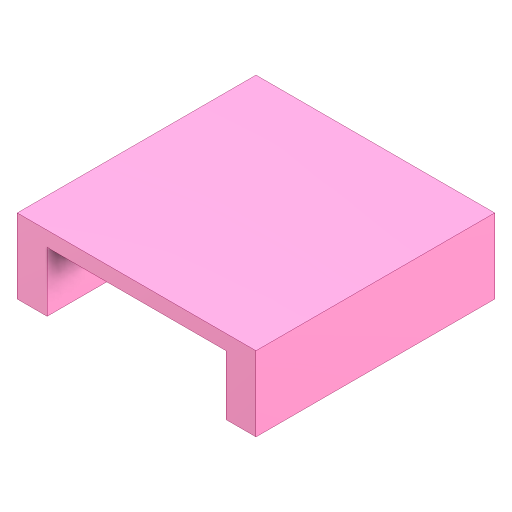
# Autodesk Inventor part: bridge_rect_final_12
Saved by Autodesk Inventor 2024 (Build 280153000, 153)
## iProperties
Created: 2023-08-28
Part Number: bridge_rect_final_12
Material: 一般
Document SubType Name: Modeling
Designer: admin
Density: 1 g/cm^3
Appearance: 平滑 - 白色
Author: admin
Autodesk Inventor part; units mm, degrees
sketch "草圖2" plane through (0, 0, 0) normal (0, 0, 1) x (1, 0, 0)
  line L0 (0, 30) -> (0, 0)
  line L1 (0, 0) -> (12, 0)
  line L2 (12, 0) -> (12, 24)
  line L3 (12, 24) -> (84, 24)
  line L4 (84, 24) -> (84, 0)
  line L5 (84, 0) -> (96, 0)
  line L6 (96, 0) -> (96, 30)
  line L7 (96, 30) -> (0, 30)
  dimension "d11" = 12
  dimension "d12" = 6
  dimension "d14" = 96
  dimension "d17" = 24
  constraints: 16 end point, 3 vertical, 2 collinear, 2 horizontal, 2 perpendicular, 1 coincident, 1 parallel
  measures "d11" distance of L0.end L1.end
  measures "d12" distance between parallel lines of L3 L7
  measures "d14" distance of L6.end L0.start
  measures "d17" distance between parallel lines of L1 L3
extrude "擠出2" add sketch "草圖2" along normal mid plane 96
ref_plane "工作平面1" through (96, 0, 48) normal (0.0872, 0, 0.9962) x (0, 1, 0)
ref_plane "工作平面2" through (96, 0, 48) normal (0.9962, 0, -0.0872) x (0, 1, 0)
ref_plane "工作平面3" through (48, 0, 48) normal (-1, 0, 0) x (0, 0, 1)
equation "\"d11\" = leg_length"
equation "\"d12\" = thickness"
equation "\"d14\" = width"
equation "\"d17\" = height"
equation "\"d15\" = length"
equation "\"width\" = 80 * ratio"
equation "\"height\" = 20 * ratio"
equation "\"length\" = width"
equation "\"leg_length\" = ratio"
equation "\"ratio\" = 1.2"
equation "\"thickness\" = 5 * ratio"
